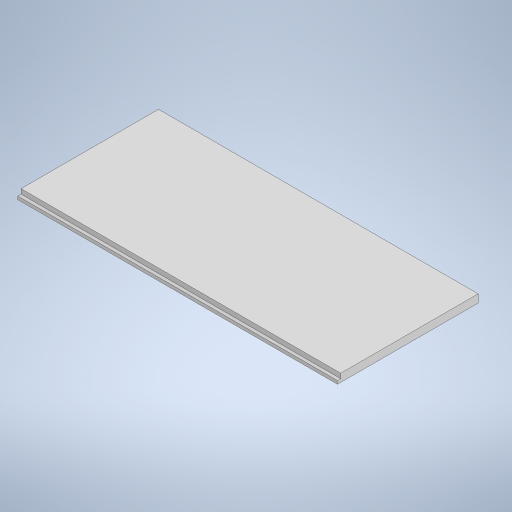
# Autodesk Inventor part: Kryt těla
Saved by Autodesk Inventor 2023.2 (Build 272271030, 271C)
## iProperties
Created: 2023-03-18
Part Number: Kryt těla
Material: Všeobecné
Document SubType Name: Modeling
Designer: jaryj
Density: 1 g/cm^3
Appearance: Výchozí
Author: jaryj
Autodesk Inventor part; units mm, degrees
ref_plane "YZ Plane" through (0, 0, 0) normal (1, 0, 0) x (0, 1, 0)
ref_plane "XZ Plane" through (0, 0, 0) normal (0, 1, 0) x (-1, 0, 0)
ref_plane "XY Plane" through (0, 0, 0) normal (0, 0, 1) x (1, 0, 0)
sketch "Náčrt1" plane through (0, 0, 0) normal (0, 1, 0) x (-1, 0, 0)
  line L0 (0, 0) -> (50, 0)
  line L1 (50, 0) -> (50, -44)
  line L2 (50, -44) -> (0, -44)
  line L3 (0, -44) -> (0, 0)
  line L4 (0, -1) -> (50, -1)
  line L5 (18, -44) -> (18, -41)
  line L6 (18, -41) -> (16, -41)
  line L7 (16, -41) -> (16, -44)
  dimension "d0" = 44
  dimension "d1" = 50
  dimension "d2" = 1
  dimension "d3" = 32
  dimension "d4" = 2
  dimension "d5" = 3
  constraints: 16 end point, 4 perpendicular, 4 point on line, 2 parallel, 1 horizontal, 1 vertical
  measures "d0" distance of L2.end L0.start
  measures "d1" distance of L1.end L2.end
  measures "d2" distance between parallel lines of L0 L4
  measures "d3" distance between parallel lines of L1 L5
  measures "d4" distance between parallel lines of L5 L7
  measures "d5" distance between parallel lines of L2 L6
extrude "Vysunutí1" add sketch "Náčrt1" along normal blind 2.5 contours L4 L1 L2 L5 L6 L7 L3 | L7 L6 L5 L2
extrude "Vysunutí2" add sketch "Náčrt1" along normal blind 1 contours L0 L1 L4 L3
extrude "Vysunutí3" add sketch "Náčrt1" against normal blind 7.5 contours L7 L6 L5 L2
sketch "Náčrt2" plane through (0, 2.5, -44) normal (0, 0, -1) x (-1, 0, 0)
  line L0 (18, -10) -> (16, -10) projected
  line L1 (18, -2.5) -> (18, -10) projected
  line L2 (16, -2.5) -> (16, -10) projected
  line L3 (16, -8) -> (16.2231, -8)
  line L4 (16.2231, -8) -> (18, -8)
  line L5 (18, -2.5) -> (18, -10) projected
  point P0 (0, -2.5)
  dimension "d12" = 2
  constraints: 4 end point, 3 point on line, 1 perpendicular
  measures "d12" distance between parallel lines of L4 L0
extrude "Vysunutí4" add sketch "Náčrt2" along normal blind 5
mirror "Zrcadlit1" about plane through (0, 0, -1) normal (1, 0, 0)
